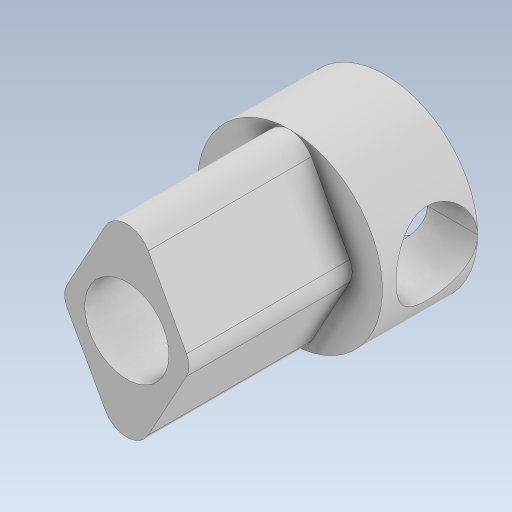
# Autodesk Inventor part: Coupling_0519
Saved by Autodesk Inventor 2023 (Build 270158000, 158)
## iProperties
Created: 2023-05-19
Part Number: Coupling_0519
Material: 一般
Document SubType Name: Modeling
Designer: JOU
Density: 1 g/cm^3
Appearance: 預設
Author: JOU
Autodesk Inventor part; units mm, degrees
ref_plane "XZ Plane" through (0, 0, 0) normal (0, 1, 0) x (-1, 0, 0)
ref_plane "XY Plane" through (0, 0, 0) normal (0, 0, 1) x (1, 0, 0)
sketch "草圖1" plane through (0, 0, 0) normal (0, 0, 1) x (1, 0, 0)
  circle A0 centre (0, 0) radius 3.4
  dimension "d0" = 6.8
  constraints: 1 centre point, 1 coincident
  measures "d0" diameter of A0
extrude "擠出1" add sketch "草圖1" along normal blind 6.5
sketch "草圖2" plane through (0, 0, 6.5) normal (0, 0, 1) x (1, 0, 0)
  circle A0 centre (0, 0) radius 1.55
  dimension "d3" = 3.1
  constraints: 1 centre point, 1 coincident
  measures "d3" diameter of A0
extrude "擠出2" cut sketch "草圖2" against normal up to surface (6.5 mm away)
ref_plane "工作平面1" through (3.4, 0, 0) normal (1, 0, 0) x (0, 1, 0)
sketch "草圖3" plane through (3.4, 0, 0) normal (1, 0, 0) x (0, 1, 0)
  circle A0 centre (0, 1.5) radius 1.5
  line L0 (0, -1.3) -> (0, 7.8) projected
  line L1 (3.4, 0) -> (-3.4, 0) projected
  point P0 (0, 0)
  dimension "d6" = 3
  constraints: 1 centre point, 1 point on line, 1 tangent
  measures "d6" diameter of A0
extrude "擠出3" cut sketch "草圖3" against normal up to surface round surface about axis through (0, 0, 6.5) along (0, 0, -1) radius 1.55 far side no
sketch "草圖4" plane through (0, 0, 6.5) normal (0, 0, 1) x (1, 0, 0)
  circle A0 centre (0, 2.5) radius 0.9
  circle A1 centre (0, -2.5) radius 0.9
  line L0 (-0.7895, 2.932) -> (-2.3938, 0)
  line L1 (-2.3938, 0) -> (-0.7895, -2.932)
  line L2 (0.7895, 2.932) -> (2.3938, 0)
  line L3 (2.3938, 0) -> (0.7895, -2.932)
  circle A2 centre (-1.5389, 0) radius 0.75
  line L4 (3.4, 0) -> (1.55, 0) projected
  circle A3 centre (1.5389, 0) radius 0.75
  line L5 (0, -4.76) -> (0, 4.76) projected
  circle A4 centre (0, 0) radius 3.4 projected
  circle A5 centre (0, 0) radius 2.1
  point P0 (0, 3.4)
  point P1 (2.1968, 0.36)
  point P2 (2.1968, -0.36)
  point P3 (0, -3.4)
  point P4 (-2.1968, -0.36)
  point P5 (-2.1968, 0.36)
  dimension "d10" = 1.8
  dimension "d13" = 1.5
  dimension "d16" = 4.2
  constraints: 9 tangent, 8 end point, 5 centre point, 4 point on circle, 3 point on line, 2 equal radius, 1 coincident, 1 parallel, 1 vertical alignment, 3 other
  measures "d10" diameter of A0
  measures "d13" diameter of A3
  measures "d16" diameter of A5
extrude "擠出4" cut sketch "草圖4" against normal blind 3 contours A0 A4 L4 L2 | A0 L0 L1 A1 A4 | A4 A1 L3 L4 | L2 L4 A3 | L3 A3 L4 | A2 L1 L0
sketch "草圖5" plane through (0, 0, 6.5) normal (0, 0, 1) x (1, 0, 0)
  arc A0 (-0.7895, -2.932) -> (0.7895, -2.932) centre (0, -2.5) ccw projected
  line L0 (0.7895, -2.932) -> (2.1968, -0.36) projected
  arc A1 (2.1968, -0.36) -> (2.1968, 0.36) centre (1.5389, 0) ccw projected
  line L1 (2.1968, 0.36) -> (0.7895, 2.932) projected
  arc A2 (0.7895, 2.932) -> (-0.7895, 2.932) centre (0, 2.5) ccw projected
  line L2 (-0.7895, 2.932) -> (-2.1968, 0.36) projected
  arc A3 (-2.1968, 0.36) -> (-2.1968, -0.36) centre (-1.5389, 0) ccw projected
  line L3 (-2.1968, -0.36) -> (-0.7895, -2.932) projected
  circle A4 centre (0, 0) radius 1.55 projected
extrude "擠出5" add sketch "草圖5" along normal blind 3
